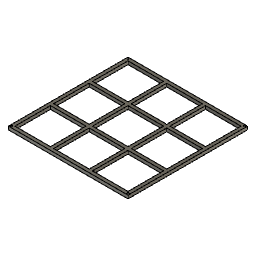
Play_board_grid v14 (Autodesk Fusion 360 design; units mm, degrees)
Autodesk Fusion 360 part; units mm, degrees
note: some values were not read from the file. Set by a fixed rule: which sketch regions a step uses.
sketch "Sketch1" plane through (0, 0, 0) normal (0, 0, 1) x (1, 0, 0)
  line L0 (110, -92.5) -> (-110, -92.5)
  line L1 (-110, -92.5) -> (-110, 92.5)
  line L2 (-110, 92.5) -> (110, 92.5)
  line L3 (110, 92.5) -> (110, -92.5)
  line L4 (110, -92.5) -> (-110, 92.5) construction
  line L5 (-110, -92.5) -> (110, 92.5) construction
  line L6 (-110, 92.5) -> (97.5144, 92.5)
  line L7 (-53.7181, -92.5) -> (-110, -92.5)
  line L8 (-110, -92.5) -> (-110, 92.5)
  line L9 (-50, 92.5) -> (-45, 92.5)
  line L10 (-45, 92.5) -> (-45, -92.5)
  line L11 (-45, -92.5) -> (-50, -92.5)
  line L12 (-50, -92.5) -> (-50, 92.5)
  line L13 (10, 92.5) -> (15, 92.5)
  line L14 (15, 92.5) -> (15, -92.5)
  line L15 (15, -92.5) -> (10, -92.5)
  line L16 (10, -92.5) -> (10, 92.5)
  line L17 (70, 92.5) -> (75, 92.5)
  line L18 (75, 92.5) -> (75, -92.5)
  line L19 (75, -92.5) -> (70, -92.5)
  line L20 (70, -92.5) -> (70, 92.5)
  line L21 (75, 42.0875) -> (75, 63.0682)
  line L22 (-110, 68) -> (-110, 42.0875)
  line L23 (75, -17.4811) -> (75, -23.4712)
  line L24 (-110, -23.4712) -> (-110, -17.4811)
  line L25 (-110, 32.5) -> (75, 32.5)
  line L26 (75, 32.5) -> (75, 27.5)
  line L27 (75, 27.5) -> (-110, 27.5)
  line L28 (-110, 27.5) -> (-110, 32.5)
  line L29 (-110, -27.5) -> (75, -27.5)
  line L30 (75, -27.5) -> (75, -32.5)
  line L31 (75, -32.5) -> (-110, -32.5)
  line L32 (-110, -32.5) -> (-110, -27.5)
  line L33 (-110, -87.5) -> (75, -87.5)
  line L34 (75, -87.5) -> (75, -92.5)
  line L35 (75, -92.5) -> (-110, -92.5)
  line L36 (-110, -92.5) -> (-110, -87.5)
  line L37 (-110, 92.5) -> (75, 92.5)
  line L38 (75, 92.5) -> (75, 87.5)
  line L39 (75, 87.5) -> (-110, 87.5)
  line L40 (-110, 87.5) -> (-110, 92.5)
  line L41 (-110, 92.5) -> (-105, 92.5)
  line L42 (-105, 92.5) -> (-105, -92.5)
  line L43 (-105, -92.5) -> (-110, -92.5)
  line L44 (-110, -92.5) -> (-110, 92.5)
  line L45 (75, 37.5) -> (110, 37.5) construction
  line L46 (75, -37.5) -> (110, -37.5) construction
  circle A0 centre (76.8705, -4.3263) radius 25 construction
  circle A1 centre (78.6242, -22.2407) radius 1.75
  circle A2 centre (76.6017, 13.6717) radius 1.75
  line L47 (75, 25.3235) -> (110, 25.3235) construction
  dimension "d3" = 220
  dimension "d5" = 5
  dimension "d6" = 5
  dimension "d8" = 5
  dimension "d10" = 55
  dimension "d11" = 55
  dimension "d13" = 5
  dimension "d16" = 5
  dimension "d17" = 5
  dimension "d18" = 5
  dimension "d19" = 55
  dimension "d20" = 55
  dimension "d22" = 55
  dimension "d23" = 5
  dimension "d24" = 55
  dimension "d25" = 55
  dimension "d26" = 55
  dimension "d27" = 50
  dimension "d32" = 3.5
  dimension "d33" = 3.5
  dimension "d34" = 18
  dimension "d35" = 18
  constraint horizontal L0
  constraint perpendicular L0 L1
  constraint parallel L0 L2
  constraint parallel L1 L3
  constraint coincident L4 origin
  constraint coincident L5 origin
  constraint horizontal L6
  constraint horizontal L7
  constraint vertical L8
  constraint coincident L0 L7.start
  constraint horizontal L9
  constraint vertical L10
  constraint horizontal L11
  constraint vertical L12
  constraint coincident L0 L10.end
  constraint coincident L2 L9.start
  constraint horizontal L13
  constraint vertical L14
  constraint horizontal L15
  constraint vertical L16
  constraint coincident L0 L14.end
  constraint coincident L2 L13.start
  constraint horizontal L17
  constraint vertical L18
  constraint horizontal L19
  constraint vertical L20
  constraint coincident L0 L18.end
  constraint coincident L2 L17.start
  constraint vertical L21
  constraint vertical L22
  constraint coincident L18 L21.end
  constraint coincident L5 L21.end
  constraint coincident L8 L22.end
  constraint vertical L23
  constraint vertical L24
  constraint coincident L18 L23.end
  constraint coincident L1 L24.end
  constraint horizontal L25
  constraint vertical L26
  constraint horizontal L27
  constraint vertical L28
  constraint coincident L18 L26.end
  constraint coincident L8 L25.start
  constraint horizontal L29
  constraint vertical L30
  constraint horizontal L31
  constraint vertical L32
  constraint coincident L18 L30.end
  constraint coincident L1 L29.start
  constraint horizontal L33
  constraint vertical L34
  constraint horizontal L35
  constraint vertical L36
  constraint coincident L8 L33.start
  constraint horizontal L37
  constraint vertical L38
  constraint horizontal L39
  constraint vertical L40
  constraint coincident L18 L38.end
  constraint horizontal L41
  constraint vertical L42
  constraint horizontal L43
  constraint vertical L44
  constraint coincident L7 L42.end
  constraint coincident L18 L45.start
  constraint coincident L3 L45.end
  constraint perpendicular L3 L45
  constraint coincident L18 L46.start
  constraint coincident L3 L46.end
  constraint perpendicular L3 L46
  constraint coincident L18 L47.start
  constraint coincident L3 L47.end
  constraint perpendicular L3 L47
  measures "d3" distance of L1.end L2.end
  measures "d5" distance of L10 L12
  measures "d6" distance of L14 L16
  measures "d8" distance of L18 L20
  measures "d10" distance of L10 L16
  measures "d11" distance of L14 L20
  measures "d13" distance of L25 L27
  measures "d16" distance of L29 L31
  measures "d17" distance of L0 L33
  measures "d18" distance of L2 L39
  measures "d19" distance of L25 L39
  measures "d20" distance of L27 L29
  measures "d22" distance of L31 L33
  measures "d23" distance of L1 L42
  measures "d24" distance of L12 L42
  measures "d25" distance of L2 L45
  measures "d26" distance of L0 L46
  measures "d27" diameter of A0
  measures "d32" diameter of A1
  measures "d33" diameter of A2
  measures "d34" distance of A0.centre A2.centre
  measures "d35" distance of A0.centre A1.centre
extrude "Extrude7" add sketch "Sketch1" along normal blind 5 contours L0 L18 L19 L20 L33 L34 L35 | L0 L14 L20 L33 L35 | L18 L20 L31 L33 | L0 L14 L15 L16 L33 L35 | L18 L20 L29 L30 L31 | L2 L6 L17 L18 L20 L37 L38 L39 | L0 L10 L16 L33 L35 | L14 L16 L31 L33 | L14 L20 L29 L31 | L18 L20 L23 L27 L29 A2 | L2 L6 L14 L20 L37 L39 | L18 L20 L21 L25 L39 | L0 L10 L11 L12 L33 L35 | L14 L16 L29 L31 | L2 L6 L13 L14 L16 L37 L39 | L0 L7 L12 L33 L35 L42 | L10 L12 L31 L33 | L10 L16 L29 L31 | L14 L16 L27 L29 | L14 L20 L25 L27 | L18 L20 L25 L26 L27 | L2 L6 L10 L16 L37 L39 | L14 L16 L25 L39 | L10 L12 L29 L31 | L14 L16 L25 L27 | L18 A2 | L2 L6 L9 L10 L12 L37 L39 | L0 L1 L7 L8 L33 L35 L36 L42 L43 L44 | L12 L29 L31 L42 | L1 L8 L31 L33 L42 L44 | L10 L12 L27 L29 | L10 L16 L25 L27 | L2 L6 L12 L37 L39 L42 | L10 L12 L25 L39 | L1 L8 L29 L31 L32 L42 L44 | L10 L12 L25 L27 | L1 L2 L6 L8 L37 L39 L40 L41 L42 L44 | L12 L25 L27 L42 | L1 L8 L24 L27 L29 L42 L44 | L1 L8 L22 L25 L39 L42 L44 | L1 L8 L25 L27 L28 L42 L44 picked at (74.9727, 13.8309)
sketch "Sketch5" plane through (0, 0, 0) normal (0, 0, 1) x (1, 0, 0)
  line L0 (-110, 92.5) -> (-105, 87.5) construction
  line L1 (-105, 92.5) -> (-110, 87.5) construction
  circle A0 centre (-107.5, 90) radius 1.4
  line L2 (70, 92.5) -> (75, 87.5) construction
  line L3 (75, 92.5) -> (70, 87.5) construction
  circle A1 centre (72.5, 90) radius 1.4
  line L4 (70, -87.5) -> (75, -92.5) construction
  line L5 (75, -87.5) -> (70, -92.5) construction
  circle A2 centre (72.5, -90) radius 1.4
  line L6 (-110, -87.5) -> (-105, -92.5) construction
  line L7 (-105, -87.5) -> (-110, -92.5) construction
  circle A3 centre (-107.5, -90) radius 1.4
  dimension "d54" = 2.8
  dimension "d55" = 2.8
  dimension "d56" = 2.8
  dimension "d57" = 2.8
  constraint midpoint L1 A0.centre
  constraint perpendicular L2 L3
  constraint midpoint L3 A1.centre
  constraint midpoint L5 A2.centre
  constraint midpoint L7 A3.centre
  measures "d54" diameter of A0
  measures "d55" diameter of A1
  measures "d56" diameter of A2
  measures "d57" diameter of A3
extrude "Extrude8" cut sketch "Sketch5" along normal through all
equation "Board_piece_lenght = 40 mm"
equation "d5 = Wall_width"
equation "d6 = Wall_width"
equation "Wall_width = 5 mm"
equation "d8 = Wall_width"
equation "d10 = Inner_sqauare"
equation "d11 = Inner_sqauare"
equation "Inner_sqauare = 55 mm"
equation "d13 = Wall_width"
equation "d16 = Wall_width"
equation "d17 = Wall_width"
equation "d18 = Wall_width"
equation "d19 = Inner_sqauare"
equation "d20 = Inner_sqauare"
equation "d22 = Inner_sqauare"
equation "d23 = Wall_width"
equation "d24 = Inner_sqauare"
equation "d25 = Inner_sqauare"
equation "d26 = Inner_sqauare"
